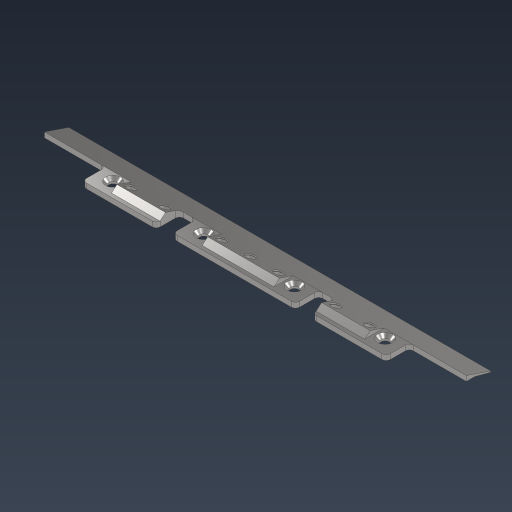
# Autodesk Inventor part: plog
Saved by Autodesk Inventor 2023 (Build 270158000, 158)
## iProperties
Created: 2024-04-10
Part Number: plog
Material: Steel, Alloy
Document SubType Name: Modeling
Designer: szymo
Density: 7.73 g/cm^3
Appearance: Semi-Polished
Mass: 133.987 g
Surface Area: 104.424 cm^2
Volume: 17.3334 cm^3
TOTAL MASS: 0.0
Author: szymo
Autodesk Inventor part; units mm, degrees
sketch "Sketch3" plane through (0, 0, 0) normal (1, 0, 0) x (0, 1, 0)
  line L0 (0, 0) -> (9, 0)
  line L1 (9, 0) -> (9, -14)
  line L2 (9, -14) -> (0, -14)
  line L3 (0, -14) -> (0, 0)
  line L4 (9, 0) -> (0, -14)
  line L5 (8, 0) -> (3.5, 0)
  line L6 (3.5, 0) -> (3.5, 15)
  line L7 (3.5, 15) -> (8, 15)
  line L8 (8, 15) -> (8, 0)
  line L9 (8.5, 0) -> (8, 0)
  line L10 (8, 0) -> (8, 4)
  point P0 (3.5, 0)
  dimension "d30" = 15
  dimension "d31" = 4.5
  dimension "d63" = 9
  dimension "d141" = 32.735
  dimension "d142" = 14
  dimension "d143" = 3.5
  dimension "d144" = 1
  constraints: 22 end point, 4 perpendicular, 3 point on line, 1 collinear
  measures "d30" distance of L5.end L6.end
  measures "d31" distance of L6.end L7.end
  measures "d63" distance of L1.end L2.end
  measures "d141" angle of L4 L3
  measures "d142" distance of L0.end L1.end
  measures "d143" distance between parallel lines of L6 L3
  measures "d144" distance from line of L8 L0.end
extrude "Extrusion2" add sketch "Sketch3" along normal blind 178 contours L0 L4 L3 | L6 L7 L8 L0
sketch "Sketch10" plane through (0, 3.5, -14) normal (0, -1, 0) x (1, 0, 0)
  line L0 (0, 14) -> (0, 26)
  line L1 (0, 26) -> (178, 26)
  line L2 (178, 14) -> (178, 26)
  line L3 (0, 14) -> (0, 18)
  line L4 (0, 18) -> (17, 18)
  line L5 (17, 18) -> (17, 26)
  line L6 (17, 26) -> (0, 26)
  line L7 (0, 26) -> (0, 18)
  line L8 (0, 18) -> (178, 18)
  line L9 (178, 26) -> (161, 26)
  line L10 (161, 26) -> (161, 18)
  line L11 (161, 18) -> (178, 18)
  line L12 (178, 18) -> (178, 26)
  line L13 (17, 26) -> (32, 26)
  line L14 (32, 26) -> (32, 18)
  line L15 (32, 18) -> (17, 18)
  line L16 (17, 18) -> (17, 26)
  line L17 (60, 26) -> (75, 26)
  line L18 (75, 26) -> (75, 18)
  line L19 (75, 18) -> (60, 18)
  line L20 (60, 18) -> (60, 26)
  line L21 (103, 26) -> (118, 26)
  line L22 (118, 26) -> (118, 18)
  line L23 (118, 18) -> (103, 18)
  line L24 (103, 18) -> (103, 26)
  line L25 (146, 26) -> (161, 26)
  line L26 (161, 26) -> (161, 18)
  line L27 (161, 18) -> (146, 18)
  line L28 (146, 18) -> (146, 26)
  line L29 (17, 26) -> (32, 18)
  line L30 (32, 26) -> (17, 18)
  line L31 (60, 26) -> (75, 18)
  line L32 (75, 26) -> (60, 18)
  line L33 (103, 26) -> (118, 18)
  line L34 (118, 26) -> (103, 18)
  line L35 (146, 26) -> (161, 18)
  line L36 (161, 26) -> (146, 18)
  line L37 (0, 14) -> (178, 14)
  line L38 (178, 26) -> (161, 26)
  line L39 (161, 26) -> (161, 33.1494)
  line L40 (161, 33.1494) -> (178, 33.1494)
  line L41 (178, 33.1494) -> (178, 26)
  line L42 (146, 26) -> (118, 26)
  line L43 (118, 26) -> (118, 37.5544)
  line L44 (118, 37.5544) -> (146, 37.5544)
  line L45 (146, 37.5544) -> (146, 26)
  line L46 (103, 26) -> (75, 26)
  line L47 (75, 26) -> (75, 36.0625)
  line L48 (75, 36.0625) -> (103, 36.0625)
  line L49 (103, 36.0625) -> (103, 26)
  line L50 (60, 26) -> (32, 26)
  line L51 (32, 26) -> (32, 34.4304)
  line L52 (32, 34.4304) -> (60, 34.4304)
  line L53 (60, 34.4304) -> (60, 26)
  line L54 (17, 26) -> (0, 26)
  line L55 (0, 26) -> (0, 37.0756)
  line L56 (0, 37.0756) -> (17, 37.0756)
  line L57 (17, 37.0756) -> (17, 26)
  point P0 (118, 26)
  point P1 (24.5, 22)
  point P2 (67.5, 22)
  point P3 (110.5, 22)
  point P4 (153.5, 22)
  dimension "d118" = 17
  dimension "d119" = 17
  dimension "d120" = 15
  dimension "d121" = 15
  dimension "d122" = 15
  dimension "d123" = 15
  dimension "d124" = 0
  dimension "d125" = 0
  dimension "d126" = 28
  dimension "d129" = 28
  dimension "d130" = 28
  constraints: 116 end point, 10 parallel, 5 horizontal, 5 perpendicular, 5 point on line, 4 midpoint
  measures "d118" distance of L6.end L5.end
  measures "d119" distance of L11.end L10.end
  measures "d120" distance of L14.end L15.end
  measures "d121" distance of L18.end L19.end
  measures "d122" distance of L22.end L23.end
  measures "d123" distance of L26.end L27.end
  measures "d124" distance between parallel lines of L5 L16
  measures "d125" distance between parallel lines of L26 L10
  measures "d126" distance between parallel lines of L22 L28
  measures "d129" distance between parallel lines of L14 L20
  measures "d130" distance between parallel lines of L18 L24
extrude "Extrusion5" cut sketch "Sketch10" against normal up to next contours L0 L1 L5 L4 | L55 L56 L57 L1 | L8 L10 L1 L2 | L14 L1 L20 L8 | L1 L39 L40 L41 | L51 L52 L53 L1 | L8 L22 L1 L28 | L18 L1 L24 L8 | L1 L43 L44 L45 | L47 L48 L49 L1
fillet "Fillet3" radius 2 8 edges at (161, 5.75, 4) (146, 5.75, 4) (118, 5.75, 4) (103, 5.75, 4) (75, 5.75, 4) (60, 5.75, 4) (32, 5.75, 4) (17, 5.75, 4)
sketch "Sketch11" plane through (0, 8, 0) normal (0, 1, 0) x (1, 0, 0)
  point P0 (0, 0)
  point P1 (24.5, -8)
  point P2 (67.5, -8)
  point P3 (110.5, -8)
  point P4 (153.5, -8)
hole "Hole5" at (24.5, 8, 8) at (67.5, 8, 8) at (110.5, 8, 8) at (153.5, 8, 8) direction (0, -1, 0) diameter 2.459 depth 8.8 thread size "M3x0.5" class "6H" standard "ISO Metric profile"
sketch "Sketch12" plane through (178, 0, 0) normal (1, 0, 0) x (0, 0, -1)
  line L0 (-4, 8) -> (-4, 3.5) projected
  line L1 (-4, 3.5) -> (0, 3.5) projected
  line L2 (0, 3.5) -> (0, 0) projected
  line L3 (0, 0) -> (14, 0) projected
  line L4 (14, 0) -> (0, 9) projected
  line L5 (0, 9) -> (0, 8) projected
  line L6 (0, 8) -> (-4, 8) projected
  line L7 (-3.1035, 5.6133) -> (13.9355, -0.1893)
  line L8 (0, 3.5) -> (7.4239, 1.5)
  line L9 (7.4239, 1.5) -> (7.5851, 1.9733)
  line L10 (-3.1035, 5.6133) -> (-4, 5.9186)
  line L11 (-4, 3.5) -> (-4, 8) projected
  dimension "d153" = 0.5
  dimension "d154" = 1.5
  constraints: 8 end point, 2 point on line, 1 collinear, 1 perpendicular, 3 other
  measures "d153" distance of L8.end L9.end
  measures "d154" distance from line of L3 L8.end
extrude "Extrusion6" cut sketch "Sketch12" against normal up to surface (178 mm away) contours L6 L5 L4 L3 L7 L10 L0 | L8 L9 L7 L3 L2
sketch "Sketch13" plane through (146, 8, 15) normal (0, 1, 0) x (1, 0, 0)
  line L0 (-69, 11) -> (-88, 11) projected
  arc A0 (-86, 9) -> (-88, 11) centre (-88, 9) ccw projected
  line L1 (-86, 9) -> (-86, 0) projected
  line L2 (-86, 0) -> (-71, 0) projected
  line L3 (-71, 0) -> (-71, 9) projected
  arc A1 (-69, 11) -> (-71, 9) centre (-69, 9) ccw projected
  circle A2 centre (-78.5, 7) radius 1.2295 projected
  line L4 (-112, 11) -> (-131, 11) projected
  arc A3 (-129, 9) -> (-131, 11) centre (-131, 9) ccw projected
  line L5 (-129, 9) -> (-129, 0) projected
  line L6 (-129, 0) -> (-114, 0) projected
  line L7 (-114, 0) -> (-114, 9) projected
  arc A4 (-112, 11) -> (-114, 9) centre (-112, 9) ccw projected
  circle A5 centre (-121.5, 7) radius 1.2295 projected
  circle A6 centre (-35.5, 7) radius 1.2295 projected
  line L8 (-26, 11) -> (-45, 11) projected
  arc A7 (-43, 9) -> (-45, 11) centre (-45, 9) ccw projected
  line L9 (-43, 9) -> (-43, 0) projected
  line L10 (-43, 0) -> (-28, 0) projected
  line L11 (-28, 0) -> (-28, 9) projected
  arc A8 (-26, 11) -> (-28, 9) centre (-26, 9) ccw projected
  line L12 (17, 11) -> (-2, 11) projected
  arc A9 (0, 9) -> (-2, 11) centre (-2, 9) ccw projected
  line L13 (0, 9) -> (0, 0) projected
  line L14 (0, 0) -> (15, 0) projected
  line L15 (15, 0) -> (15, 9) projected
  arc A10 (17, 11) -> (15, 9) centre (17, 9) ccw projected
  circle A11 centre (7.5, 7) radius 1.2295 projected
  line L16 (0, 9) -> (0, 11)
  line L17 (17, 11) -> (-2, 11) projected
  line L18 (-28, 9) -> (-28, 11.1215)
  line L19 (-43, 9) -> (-43, 11)
  arc A12 (-69, 11) -> (-71, 9) centre (-69, 9) ccw projected
  line L20 (-71, 9) -> (-71, 11.1215)
  line L21 (-86, 9) -> (-86, 11)
  line L22 (-114, 9) -> (-114, 11)
  arc A13 (-129, 9) -> (-131, 11) centre (-131, 9) ccw projected
  line L23 (-129, 9) -> (-129, 11.1215)
  line L24 (15, 9) -> (15, 0) projected
  line L25 (15, 9) -> (15, 11)
  point P0 (-146, 15)
  point P1 (-71, 11)
  point P2 (-28, 11)
  point P3 (0, 11)
  point P4 (-129, 11)
  constraints: 16 end point, 7 tangent, 6 perpendicular, 5 point on line, 1 parallel, 1 point on circle, 1 vertical
extrude "Extrusion7" cut sketch "Sketch13" against normal through all contours L21 A0 L0 | L0 A1 L20 | A4 L22 L4 | L23 A3 L4 | A6 | L19 A7 L8 | L8 A8 L18 | A10 L25 L12 | L16 A9 L12
sketch "Sketch14" plane through (103, 8, 15) normal (0, 1, 0) x (1, 0, 0)
  line L0 (43, 11) -> (43, 0) projected
  line L1 (43, 0) -> (58, 0) projected
  line L2 (58, 0) -> (58, 11) projected
  line L3 (58, 11) -> (43, 11) projected
  circle A0 centre (50.5, 7) radius 1.2295 projected
  line L4 (0, 11) -> (0, 0) projected
  line L5 (0, 0) -> (15, 0) projected
  line L6 (15, 0) -> (15, 11) projected
  line L7 (15, 11) -> (0, 11) projected
  circle A1 centre (7.5, 7) radius 1.2295 projected
  line L8 (-43, 11) -> (-43, 0) projected
  line L9 (-43, 0) -> (-28, 0) projected
  line L10 (-28, 0) -> (-28, 11) projected
  line L11 (-28, 11) -> (-43, 11) projected
  circle A2 centre (-35.5, 7) radius 1.2295 projected
  circle A3 centre (-78.5, 7) radius 1.2295 projected
  line L12 (-71, 0) -> (-71, 11) projected
  line L13 (58, 11) -> (43, 11) projected
  line L14 (-86, 11) -> (-86, 0) projected
  line L15 (-86, 0) -> (-71, 0) projected
  line L16 (0, 11) -> (-28, 11) projected
  line L17 (0, 11) -> (-28, 11)
  line L18 (0, 0) -> (15, 0) projected
  line L19 (0, 0) -> (-28, 0)
  line L20 (-86, 0) -> (-71, 0) projected
  line L21 (-43, 11) -> (-71, 11) projected
  line L22 (-71, 0) -> (-51, 0)
  line L23 (-51, 0) -> (-51, 11)
  line L24 (-51, 11) -> (-71, 11)
  line L25 (-71, 11) -> (-71, 0)
  line L26 (43, 0) -> (43, 11) projected
  line L27 (43, 11) -> (15, 11) projected
  line L28 (43, 0) -> (23, 0)
  line L29 (23, 0) -> (23, 11)
  line L30 (23, 11) -> (43, 11)
  line L31 (43, 11) -> (43, 0)
  line L32 (16.5, 4.4498) -> (16.5, 7.75)
  line L33 (21.5, 4.4498) -> (21.5, 7.75)
  line L34 (43, 11) -> (43, 0) projected
  line L35 (43, 0) -> (58, 0) projected
  line L36 (58, 0) -> (58, 11) projected
  line L37 (-43, 11) -> (-43, 0) projected
  line L38 (-43, 0) -> (-28, 0) projected
  line L39 (-28, 0) -> (-28, 11) projected
  line L40 (-28, 11) -> (-43, 11) projected
  line L41 (-71, 11) -> (-86, 11) projected
  line L42 (15, 0) -> (15, 11) projected
  line L43 (15, 11) -> (0, 11) projected
  line L44 (0, 11) -> (0, 0) projected
  line L45 (0, 0) -> (15, 0) projected
  line L46 (-86, 11) -> (-86, 0) projected
  line L47 (-86, 0) -> (-71, 0) projected
  line L48 (-71, 0) -> (-71, 11) projected
  line L49 (-71, 11) -> (-86, 11) projected
  line L50 (15, 0) -> (15, 11) projected
  line L51 (15, 11) -> (0, 11) projected
  line L52 (0, 11) -> (0, 0) projected
  line L53 (0, 0) -> (15, 0) projected
  line L54 (-28, 0) -> (-28, 11) projected
  line L55 (-28, 11) -> (-43, 11) projected
  line L56 (-43, 11) -> (-43, 0) projected
  line L57 (-43, 0) -> (-28, 0) projected
  point P0 (-103, 15)
  dimension "d160" = 8
  dimension "d161" = 8
  constraints: 24 end point, 4 parallel, 2 collinear, 2 horizontal, 2 perpendicular, 2 point on line, 4 other
  measures "d160" distance between parallel lines of L29 L6
  measures "d161" distance between parallel lines of L8 L23
extrude "Extrusion8" add sketch "Sketch14" against normal up to surface (4.5 mm away) contours L0 L28 L29 L27 | L4 L19 L10 L16 | L12 L21 L23 L22
sketch "Sketch15" plane through (178, 0, 0) normal (1, 0, 0) x (0, 0, -1)
  line L0 (0, 3.5) -> (7.4239, 1.5) projected
  line L1 (7.4239, 1.5) -> (7.5851, 1.9733) projected
  line L2 (7.5851, 1.9733) -> (-4, 5.9186) projected
  line L3 (-4, 5.9186) -> (-4, 3.5) projected
  line L4 (-4, 3.5) -> (0, 3.5) projected
  line L5 (-6, 3.5) -> (-4, 3.5) projected
  line L6 (-4, 3.5) -> (-4, 5.9186) projected
  line L7 (-4, 5.9186) -> (-4, 8) projected
  line L8 (-4, 8) -> (-6, 8) projected
  line L9 (-6, 8) -> (-6, 3.5) projected
  line L10 (-15, 8) -> (-4, 8) projected
  line L11 (-15, 3.5) -> (-15, 8) projected
  line L12 (-4, 3.5) -> (-15, 3.5) projected
  line L13 (-4, 5.9186) -> (-4, 8) projected
  line L14 (-4, 5.9186) -> (-15, 5.9186)
  line L15 (-15, 8) -> (-15, 3.5) projected
  line L16 (-4, 5.9186) -> (-4, 3.5) projected
  line L17 (-4, 8) -> (-4, 5.9186) projected
  point P0 (0, 0)
  constraints: 2 end point, 1 perpendicular, 1 point on line
extrude "Extrusion9" cut sketch "Sketch15" against normal through all contours L14 L9 L8 L7 | L14 L11 L10 L9
sketch "Sketch16" plane through (0, 0, 0) normal (-1, 0, 0) x (0, 0, 1)
  line L0 (-7.4239, 1.5) -> (0, 3.5) projected
  line L1 (4, 3.5) -> (0, 3.5) projected
  line L2 (4, 3.5) -> (4, 5.9186) projected
  line L3 (4, 5.9186) -> (-7.5851, 1.9733) projected
  line L4 (-7.5851, 1.9733) -> (-7.4239, 1.5) projected
  point P0 (0, 0)
ref_plane "Work Plane1" through (-12, -0.1893, -14) normal (-1, 0, 0) x (0, 0.3223679, 0.9466145)
extrude "Extrusion10" add sketch "Sketch16" along normal up to surface (12 mm away)
sketch "Sketch17" plane through (178, 0, 0) normal (1, 0, 0) x (0, 0, -1)
  line L0 (0, 3.5) -> (7.4239, 1.5) projected
  line L1 (7.4239, 1.5) -> (7.5851, 1.9733) projected
  line L2 (7.5851, 1.9733) -> (-4, 5.9186) projected
  line L3 (-4, 5.9186) -> (-4, 3.5) projected
  line L4 (-4, 3.5) -> (0, 3.5) projected
  point P0 (0, 0)
ref_plane "Work Plane2" through (188, -0.1893, -14) normal (1, 0, 0) x (0, 0.9466145, -0.3223679)
extrude "Extrusion11" add sketch "Sketch17" along normal up to surface (10 mm away)
sketch "Sketch18" plane through (188, 3.5, 4) normal (1, 0, 0) x (0, 0, -1)
  line L0 (11.5851, -1.5267) -> (0, 2.4186) projected
  line L1 (0, 2.4186) -> (-6.6263, 4.6752)
  line L2 (0, 2.4186) -> (-2, 2.4186) projected
  line L3 (-2, 2.4186) -> (-2, 0) projected
  line L4 (-2, 0) -> (0, 0) projected
  line L5 (0, 0) -> (0, 2.4186) projected
  line L6 (0, 2.4186) -> (-11, 2.4186) projected
  line L7 (-11, 0) -> (-11, 2.4186) projected
  line L8 (0, 0) -> (-11, 0) projected
  line L9 (-6.6263, 4.6752) -> (-9.2045, 2.4186)
  line L10 (0, 2.4186) -> (0, 0) projected
  point P0 (4, -3.5)
  point P1 (0, 2.4186)
  point P2 (-2, 2.4186)
  dimension "d170" = 7
  dimension "d171" = 120
  constraints: 4 end point, 1 collinear, 1 point on line
  measures "d170" distance of L0.end L1.end
  measures "d171" angle of L1 L9
extrude "Extrusion12" add sketch "Sketch18" against normal up to surface (171 mm away) contours L2 L6 L9 L1
sketch "Sketch19" plane through (118, 5.9186, 13.2045) normal (0, -1, 0) x (1, 0, 0)
  line L0 (-58, 0) -> (-58, -9.2045) projected
  line L1 (-58, 0) -> (-66, 0) projected
  line L2 (-66, -9.2045) -> (-66, 0) projected
  line L3 (-58, -9.2045) -> (-66, -9.2045) projected
  line L4 (70, -2.5782) -> (-101, -2.5782) projected
  line L5 (8, 0) -> (8, -9.2045) projected
  line L6 (8, 0) -> (0, 0) projected
  line L7 (0, -9.2045) -> (0, 0) projected
  line L8 (8, -9.2045) -> (0, -9.2045) projected
  line L9 (43, -9.2045) -> (43, 0) projected
  line L10 (70, -9.2045) -> (43, -9.2045) projected
  line L11 (70, 0) -> (70, -9.2045) projected
  line L12 (70, 0) -> (43, 0) projected
  point P0 (-118, -13.2045)
  point P1 (43, -2.5782)
extrude "Extrusion13" cut sketch "Sketch19" against normal through all
ref_plane "Work Plane3" through (60, 20.5, 15) normal (0, -1, 0) x (1, 0, 0)
sketch "Sketch20" plane through (60, 20.5, 15) normal (0, -1, 0) x (1, 0, 0)
  line L0 (66, -11) -> (58, -11) projected
  line L1 (58, -11) -> (58, 0) projected
  line L2 (0, 0) -> (58, 0) projected
  line L3 (0, 0) -> (0, -11) projected
  line L4 (0, -11) -> (-8, -11) projected
  line L5 (-8, 0) -> (-8, -11) projected
  line L6 (-43, 0) -> (-8, 0) projected
  line L7 (-43, 0) -> (-43, -11) projected
  line L8 (-43, -11) -> (-72, -11) projected
  line L9 (-72, -11) -> (-72, -15) projected
  line L10 (128, -15) -> (-72, -15) projected
  line L11 (128, -15) -> (128, -11) projected
  line L12 (128, -11) -> (101, -11) projected
  line L13 (101, -11) -> (101, 0) projected
  line L14 (66, 0) -> (101, 0) projected
  line L15 (66, -11) -> (66, 0) projected
  circle A0 centre (50.5, -7) radius 1.2295 projected
  circle A1 centre (-35.5, -7) radius 1.2295 projected
  circle A2 centre (7.5, -7) radius 1.2295 projected
  circle A3 centre (93.5, -7) radius 1.2295 projected
  line L16 (101, 0) -> (89, 0)
  line L17 (89, 0) -> (89, -11)
  line L18 (89, -11) -> (101, -11)
  line L19 (101, -11) -> (101, 0)
  line L20 (-43, 0) -> (-31, 0)
  line L21 (-31, 0) -> (-31, -11)
  line L22 (-31, -11) -> (-43, -11)
  line L23 (-43, -11) -> (-43, 0)
  line L24 (0, 0) -> (12, 0)
  line L25 (12, 0) -> (12, -11)
  line L26 (12, -11) -> (0, -11)
  line L27 (0, -11) -> (0, 0)
  line L28 (58, 0) -> (46, 0)
  line L29 (46, 0) -> (46, -11)
  line L30 (46, -11) -> (58, -11)
  line L31 (58, -11) -> (58, 0)
  circle A4 centre (50.5, -7) radius 3.5
  circle A5 centre (7.5, -7) radius 1.2295 projected
  circle A6 centre (7.5, -7) radius 3.5
  circle A7 centre (93.5, -7) radius 1.2295 projected
  circle A8 centre (93.5, -7) radius 3.5
  circle A9 centre (-35.5, -7) radius 1.2295 projected
  circle A10 centre (-35.5, -7) radius 3.5
  point P0 (-60, -15)
  point P1 (-31, 0)
  point P2 (12, 0)
  point P3 (46, 0)
  point P4 (89, 0)
  dimension "d177" = 12
  dimension "d178" = 11
  dimension "d179" = 12
  dimension "d180" = 11
  dimension "d181" = 12
  dimension "d182" = 11
  dimension "d183" = 12
  dimension "d184" = 11
  dimension "d185" = 7
  dimension "d186" = 7
  dimension "d187" = 7
  dimension "d188" = 7
  constraints: 32 end point, 8 parallel, 4 centre point, 4 coincident, 4 horizontal, 4 perpendicular
  measures "d177" distance of L18.end L17.end
  measures "d178" distance of L17.end L16.end
  measures "d179" distance of L21.end L22.end
  measures "d180" distance of L20.end L21.end
  measures "d181" distance of L25.end L26.end
  measures "d182" distance of L24.end L25.end
  measures "d183" distance of L30.end L29.end
  measures "d184" distance of L29.end L28.end
  measures "d185" diameter of A4
  measures "d186" diameter of A6
  measures "d187" diameter of A8
  measures "d188" diameter of A10
extrude "Extrusion14" cut sketch "Sketch20" along normal up to surface (14.5814 mm away) contours L30 L29 L2 L1 | L14 L13 L18 L17 | L25 L26 L3 L2 | L21 L22 L7 L6 | A0 | A1 | A2 | A3 | A4 | A6 | A8 | A10
sketch "Sketch21" plane through (118, 5.9186, 4) normal (0, 0.9466145, -0.3223679) x (1, 0, 0)
  line L0 (-58, 0) -> (-46, 0) projected
  line L1 (-46, 0) -> (-46, -7) projected
  line L2 (-12, -7) -> (-46, -7) projected
  line L3 (-12, -7) -> (-12, 0) projected
  line L4 (-12, 0) -> (0, 0) projected
  line L5 (8, 0) -> (0, 0) projected
  line L6 (8, 0) -> (8, -7) projected
  line L7 (31, -7) -> (8, -7) projected
  line L8 (31, -7) -> (31, 0) projected
  line L9 (31, 0) -> (43, 0) projected
  line L10 (70, 0) -> (43, 0) projected
  line L11 (70, 0) -> (70, 12.2384) projected
  line L12 (70, 12.2384) -> (-130, 12.2384) projected
  line L13 (-130, 12.2384) -> (-130, 0) projected
  line L14 (-101, 0) -> (-130, 0) projected
  line L15 (-101, 0) -> (-89, 0) projected
  line L16 (-89, 0) -> (-89, -7) projected
  line L17 (-66, -7) -> (-89, -7) projected
  line L18 (-66, -7) -> (-66, 0) projected
  line L19 (-58, 0) -> (-66, 0) projected
  line L20 (31, 0) -> (-89, 0)
  circle A0 centre (-15.5, -3.5) radius 3.5
  circle A1 centre (-42.5, -3.5) radius 3.5
  circle A2 centre (27.5, -3.5) radius 3.5
  circle A3 centre (-85.5, -3.5) radius 3.5
  circle A4 centre (11.5, -3.5) radius 3.5
  circle A5 centre (-29, -3.5) radius 3.5
  circle A6 centre (-69.5, -3.5) radius 3.5
  point P0 (-118, 5.6944)
  dimension "d191" = 13.5
  dimension "d192" = 13.5
  constraints: 20 tangent, 7 centre point, 7 coincident, 2 end point, 1 collinear
  measures "d191" distance of A5.centre A1.centre
  measures "d192" distance of A0.centre A5.centre
hole "Hole6" at (102.5, 7.0469, 7.3132) at (89, 7.0469, 7.3132) at (75.5, 7.0469, 7.3132) at (48.5, 7.0469, 7.3132) at (32.5, 7.0469, 7.3132) at (145.5, 7.0469, 7.3132) at (129.5, 7.0469, 7.3132) direction (0, -0.9466145, 0.3223679) diameter 4 depth 3 counterbore diameter 4.5 counterbore depth 0.5
sketch "Sketch22" plane through (60, 5.9186, 15) normal (0, 1, 0) x (1, 0, 0)
  circle A0 centre (-35.5, 7) radius 1.2295 projected
  circle A1 centre (7.5, 7) radius 1.2295 projected
  circle A2 centre (50.5, 7) radius 1.2295 projected
  circle A3 centre (93.5, 7) radius 1.2295 projected
  point P0 (-60, 15)
hole "Hole7" at (24.5, 5.9186, 8) at (67.5, 5.9186, 8) at (110.5, 5.9186, 8) at (153.5, 5.9186, 8) direction (0, -1, 0) diameter 4 depth 3 countersink diameter 7 countersink angle 90
fillet "Fillet4" radius 2 12 edges at (161, 4.7093, 4) (161, 4.7093, 15) (126, 4.7093, 15) (126, 4.7093, 4) (118, 4.7093, 4) (118, 4.7093, 15) (60, 4.7093, 15) (60, 4.7093, 4) (52, 4.7093, 4) (52, 4.7093, 15) (17, 4.7093, 4) (17, 4.7093, 15)
equation "\"d126\" = d130"
equation "\"d129\" = d130"
body "Solid2"
